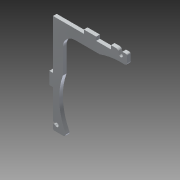
# Autodesk Inventor part: OpenROV 2_3 Dev Tube Brace
Saved by Autodesk Inventor 2015 (Build 190159000, 159)
## iProperties
Created: 2011-09-22
Part Number: OpenROV 2_3 Dev Tube Brace
Document SubType Name: Modeling
Designer: user
Density: 1 g/cm^3
Material: Generic
Appearance: Default
Author: user
Autodesk Inventor part; units mm, degrees
ref_plane "YZ Plane" through (0, 0, 0) normal (1, 0, 0) x (0, 1, 0)
ref_plane "XZ Plane" through (0, 0, 0) normal (0, 1, 0) x (-1, 0, 0)
ref_plane "XY Plane" through (0, 0, 0) normal (0, 0, 1) x (1, 0, 0)
sketch "Sketch2" plane through (0, 0, 0) normal (1, 0, 0) x (0, 1, 0)
  line L0 (55, 30) -> (58, 30)
  line L1 (58, 30) -> (58, 20)
  line L2 (58, 20) -> (55, 20)
  line L3 (15, 55) -> (15, 58)
  line L4 (15, 58) -> (5, 58)
  line L5 (5, 58) -> (5, 55)
  line L6 (55, 30) -> (55, 55)
  line L7 (15, 55) -> (55, 55)
  line L8 (55, 20) -> (55, 8)
  line L9 (55, 8) -> (58, 8)
  arc A0 (54.5719, 1.4376) -> (56.0607, -1.0607) centre (55, 0) ccw
  line L10 (57, -5) -> (51.9134, -5)
  line L11 (56.5709, 2.033) -> (54.5719, 1.4376)
  line L12 (56.2929, -0.8284) -> (56.0607, -1.0607)
  line L13 (58, 8) -> (58, 3.9497)
  line L14 (58, -1.5355) -> (58, -4)
  arc A1 (56.5709, 2.033) -> (58, 3.9497) centre (56, 3.9497) ccw
  arc A2 (58, -1.5355) -> (56.2929, -0.8284) centre (57, -1.5355) ccw
  arc A3 (57, -5) -> (58, -4) centre (57, -4) ccw
  line L15 (-25, 54) -> (-25, 46.6369)
  arc A4 (-20.9, 53.2) -> (-18.701, 52.75) centre (-20, 52) ccw
  line L16 (-20.9, 53.2) -> (-20.9, 53.2)
  line L17 (-19.134, 53.5) -> (-18.701, 52.75)
  line L18 (5, 55) -> (-18.2679, 55)
  line L19 (-21.5, 55) -> (-24, 55)
  arc A5 (-18.2679, 55) -> (-19.134, 53.5) centre (-18.2679, 54) ccw
  arc A6 (-25, 46.6369) -> (-22.1154, 44.8432) centre (-23, 46.6369) ccw
  arc A7 (-24, 55) -> (-25, 54) centre (-24, 54) ccw
  arc A8 (-20.9, 53.2) -> (-21.5, 55) centre (-21.5, 54) ccw
  arc A9 (49.9167, -2.8846) -> (47.1154, 16.7374) centre (0, 0) ccw
  arc A10 (16.7374, 47.1154) -> (-22.1154, 44.8432) centre (0, 0) ccw
  line L20 (47, 17.4069) -> (47, 37)
  line L21 (17.4069, 47) -> (37, 47)
  arc A11 (47, 37) -> (37, 47) centre (37, 37) ccw
  arc A12 (49.9167, -2.8846) -> (51.9134, -5) centre (51.9134, -3) ccw
  arc A13 (16.7374, 47.1154) -> (17.4069, 47) centre (17.4069, 49) ccw
  arc A14 (47, 17.4069) -> (47.1154, 16.7374) centre (49, 17.4069) ccw
  point P0 (-25, 43.3013)
  point P1 (58, -5)
  point P2 (-25, 55)
  point P3 (49.7494, -5)
  point P4 (49.7494, -5)
  point P5 (17.0587, 47)
  point P6 (47, 17.0587)
  dimension "d5" = 10
  dimension "d6" = 10
  dimension "d13" = 40
  dimension "d14" = 25
  dimension "d15" = 3
  dimension "d16" = 3
  dimension "d22" = 55
  dimension "d23" = 55
  dimension "d43" = 12
  dimension "d44" = 3
  dimension "d46" = 3
  dimension "d48" = 3
  dimension "d53" = 2
  dimension "d54" = 1
  dimension "d57" = 80
  dimension "d58" = 3
  dimension "d59" = 5
  dimension "d61" = 3
  dimension "d64" = 1
  dimension "d65" = 2
  dimension "d66" = 1
  dimension "d67" = 3
  dimension "d75" = 4.0503
  dimension "d76" = 60
  dimension "d78" = 5
  dimension "d79" = 3
  dimension "d87" = 60
  dimension "d92" = 8
  dimension "d93" = 50
  dimension "d94" = 50
  dimension "d95" = 8
  dimension "d96" = 10
  dimension "d97" = 2
  dimension "d98" = 2
  constraints: 44 end point, 33 point on circle, 25 tangent, 15 centre point, 11 perpendicular, 9 point on line, 4 parallel, 3 equal radius, 2 coincident, 1 horizontal
  measures "d5" distance of L0.end L1.end
  measures "d6" distance of L3.end L4.end
  measures "d13" distance between parallel lines of L6 L3
  measures "d14" distance between parallel lines of L7 L0
  measures "d15" distance between parallel lines of L6 L1
  measures "d16" distance between parallel lines of L7 L4
  measures "d22" horizontal distance of point (0, 0) L6.end
  measures "d23" distance from line of L6 point (0, 0)
  measures "d43" distance of L2.end L8.end
  measures "d44" distance of L8.end L9.end
  measures "d46" diameter of A0
  measures "d48" distance of L1.end L2.end
  measures "d53" radius of A1
  measures "d54" radius of A2
  measures "d57" distance from line of point (-25, 55) L6
  measures "d58" diameter of A4
  measures "d59" distance from line of L15 A4.centre
  measures "d61" distance from line of L13 A0.centre
  measures "d64" radius of A5
  measures "d65" radius of A6
  measures "d66" radius of A7
  measures "d67" distance of L4.end L5.end
  measures "d75" distance of L9.end L13.end
  measures "d76" distance between parallel lines of L10 L7
  measures "d78" distance from line of L10 A0.centre
  measures "d79" distance from line of L19 A4.centre
  measures "d87" angle of L17 L18
  measures "d92" distance between parallel lines of L21 L7
  measures "d93" radius of A10
  measures "d94" radius of A9
  measures "d95" distance between parallel lines of L6 L20
  measures "d96" radius of A11
  measures "d97" radius of A12
  measures "d98" radius of A13
extrude "Extrusion3" add sketch "Sketch2" along normal blind 3
body "Solid3"
